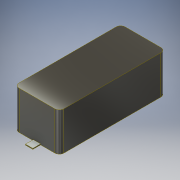
# Autodesk Inventor part: HC49_XTAL
Saved by Autodesk Inventor 2016 (Build 200138000, 138)
## iProperties
Created: 2016-09-23
Part Number: HC49_XTAL
Material: Generic
Document SubType Name: Modeling
Designer: jfixelle
Density: 1 g/cm^3
Appearance: Silver
Author: jfixelle
Autodesk Inventor part; units mm, degrees
ref_plane "YZ Plane" through (0, 0, 0) normal (1, 0, 0) x (0, 1, 0)
ref_plane "XZ Plane" through (0, 0, 0) normal (0, 1, 0) x (-1, 0, 0)
ref_plane "XY Plane" through (0, 0, 0) normal (0, 0, 1) x (1, 0, 0)
sketch "Sketch1" plane through (0, 0, 0) normal (0, 1, 0) x (-1, 0, 0)
  line L0 (2.45, 5.8) -> (-2.45, 5.8)
  line L1 (-2.45, 5.8) -> (-2.45, -5.8)
  line L2 (-2.45, -5.8) -> (2.45, -5.8)
  line L3 (2.45, -5.8) -> (2.45, 5.8)
  point P0 (0, 0)
  dimension "d0" = 11.6
  dimension "d1" = 5.8
  dimension "d2" = 4.9
  dimension "d3" = 2.45
  constraints: 8 end point, 2 parallel, 1 horizontal, 1 perpendicular
  measures "d0" distance of L2.end L0.start
  measures "d1" distance from line of point (0, 0) L2
  measures "d2" distance of L1.end L2.end
  measures "d3" distance from line of point (0, 0) L3
extrude "Extrusion1" add sketch "Sketch1" along normal blind 4.2
fillet "Fillet1" radius 0.5 4 edges at (2.45, 2.1, 5.8) (-2.45, 2.1, 5.8) (2.45, 2.1, -5.8) (-2.45, 2.1, -5.8)
sketch "Sketch2" plane through (0, 0, 0) normal (0, -1, 0) x (1, 0, 0)
  line L0 (0.4, 6.65) -> (-0.4, 6.65)
  line L1 (-0.4, 6.65) -> (-0.4, 2.4)
  line L2 (-0.4, 2.4) -> (0.4, 2.4)
  line L3 (0.4, 2.4) -> (0.4, 6.65)
  line L4 (0.4, -2.4) -> (-0.4, -2.4)
  line L5 (-0.4, -2.4) -> (-0.4, -6.65)
  line L6 (-0.4, -6.65) -> (0.4, -6.65)
  line L7 (0.4, -6.65) -> (0.4, -2.4)
  point P0 (0, 0)
  dimension "d7" = 13.3
  dimension "d9" = 4.8
  dimension "d10" = 2.4
  dimension "d11" = 6.65
  dimension "d12" = 0.8
  dimension "d13" = 0.8
  dimension "d14" = 0.4
  dimension "d15" = 0.4
  constraints: 16 end point, 4 parallel, 2 horizontal, 2 perpendicular
  measures "d7" distance between parallel lines of L0 L6
  measures "d9" distance between parallel lines of L4 L2
  measures "d10" distance from line of point (0, 0) L4
  measures "d11" distance from line of point (0, 0) L6
  measures "d12" distance of L4.start L4.end
  measures "d13" distance of L1.end L2.end
  measures "d14" distance from line of point (0, 0) L3
  measures "d15" distance from line of point (0, 0) L7
extrude "Extrusion2" add sketch "Sketch2" against normal blind 0.1
body "Solid1"
